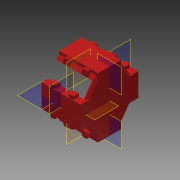
# Autodesk Inventor part: ButtConnector
Saved by Autodesk Inventor 2015 (Build 190159000, 159)
## iProperties
Created: 2015-03-02
Part Number: ButtConnector
Material: Generic
Document SubType Name: Modeling
Designer: Henke
Density: 1 g/cm^3
Appearance: Light Red
Author: Henke
Autodesk Inventor part; units mm, degrees
ref_plane "YZ Plane" through (0, 0, 0) normal (1, 0, 0) x (0, 1, 0)
ref_plane "XZ Plane" through (0, 0, 0) normal (0, 1, 0) x (-1, 0, 0)
ref_plane "XY Plane" through (0, 0, 0) normal (0, 0, 1) x (1, 0, 0)
sketch "Sketch1" plane through (0, 0, 0) normal (0, 0, 1) x (1, 0, 0)
  line L0 (0, 0) -> (35.7, 0)
  line L1 (35.7, 0) -> (35.7, 21.1)
  line L2 (35.7, 21.1) -> (0, 21.1)
  line L3 (0, 21.1) -> (0, 0)
  dimension "d0" = 35.7
  dimension "d1" = 21.1
  constraints: 8 end point, 2 parallel, 1 horizontal, 1 perpendicular
  measures "d0" distance of L1.end L2.end
  measures "d1" distance of L2.end L0.start
extrude "Extrusion1" add sketch "Sketch1" along normal blind 6
sketch "Sketch3" plane through (0, 21.1, 0) normal (0, 1, 0) x (1, 0, 0)
  line L0 (0, 0) -> (35.7, 0) projected
  line L1 (9.35, 0) -> (6.85, -1.05)
  line L2 (6.85, -1.05) -> (6.85, -5.55)
  line L3 (11.85, -5.55) -> (11.85, -1.05)
  line L4 (11.85, -1.05) -> (9.35, 0)
  line L5 (17.85, 0) -> (17.85, -6) construction
  line L6 (6.85, -5.55) -> (11.85, -5.55)
  line L7 (0, -6) -> (35.7, -6) projected
  dimension "d4" = 4.5
  dimension "d5" = 5
  dimension "d6" = 8.5
  dimension "d9" = 5.55
  constraints: 12 end point, 2 equal length, 2 midpoint, 2 vertical, 1 parallel, 1 point on line
  measures "d4" distance of L1.end L2.end
  measures "d5" distance between parallel lines of L3 L2
  measures "d6" distance from line of L5 L1.start
  measures "d9" distance from line of L6 L1.start
extrude "Extrusion2" add sketch "Sketch3" along normal blind 2.75
ref_plane "Work Plane1" through (17.85, 0, 6) normal (1, 0, 0) x (0, 1, 0)
mirror "Mirror1" about plane through (17.85, 0, 6) normal (1, 0, 0) of "Extrusion2"
ref_plane "Work Plane2" through (35.7, 10.55, 6) normal (0, 1, 0) x (-1, 0, 0)
mirror "Mirror2" about plane through (35.7, 10.55, 6) normal (0, 1, 0) of "Extrusion2", "Mirror1"
sketch "Sketch4" plane through (0, 0, 6) normal (0, 0, 1) x (1, 0, 0)
  line L0 (35.7, 21.1) -> (0, 21.1) projected
  line L1 (35.7, 0) -> (32.7, 0)
  line L2 (32.7, 0) -> (32.7, 21.1)
  line L3 (32.7, 21.1) -> (35.7, 21.1)
  line L4 (35.7, 21.1) -> (35.7, 0)
  point P0 (0, 0)
  dimension "d10" = 3
  constraints: 8 end point, 2 parallel, 1 horizontal, 1 perpendicular, 1 point on line
  measures "d10" distance between parallel lines of L4 L2
extrude "Extrusion3" add sketch "Sketch4" along normal blind 21.5
sketch "Sketch6" plane through (0, 0, 6) normal (0, 0, 1) x (1, 0, 0)
  line L0 (32.7, 0) -> (32.7, 21.1) projected
  line L1 (0, 0) -> (32.7, 0)
  line L2 (32.7, 0) -> (32.7, 3)
  line L3 (32.7, 3) -> (0, 3)
  line L4 (0, 3) -> (0, 0)
  line L5 (0, 21.1) -> (32.7, 21.1)
  line L6 (32.7, 21.1) -> (32.7, 18.1)
  line L7 (32.7, 18.1) -> (0, 18.1)
  line L8 (0, 18.1) -> (0, 21.1)
  dimension "d13" = 3
  dimension "d14" = 3
  constraints: 16 end point, 4 parallel, 2 horizontal, 2 perpendicular, 2 point on line
  measures "d13" distance of L7.end L5.start
  measures "d14" distance of L3.end L1.start
mirror "Mirror3" about plane through (34.2, 10.55, 27.5) normal (0, 0, 1) of "Extrusion1", "Extrusion2", "Mirror1", "Mirror2", "Extrusion3"
ref_plane "Work Plane5" through (32.7, 0, 27.5) normal (0, 0, 1) x (1, 0, 0)
sketch "Sketch7" plane through (0, 0, 0) normal (0, -1, 0) x (1, 0, 0)
  line L0 (35.7, 0) -> (35.7, 55) projected
  line L1 (32.7, 6) -> (32.7, 49) projected
  line L2 (35.7, 16.95) -> (32.7, 16.95)
  line L3 (32.7, 16.95) -> (32.7, 38.05)
  line L4 (32.7, 38.05) -> (35.7, 38.05)
  line L5 (35.7, 38.05) -> (35.7, 16.95)
  line L6 (32.7, 6) -> (32.7, 49) projected
  point P0 (0, 0)
  point P1 (32.7, 27.5)
  point P2 (32.7, 27.5)
  dimension "d15" = 21.1
  constraints: 8 end point, 2 midpoint, 2 parallel, 2 point on line, 1 coincident, 1 horizontal, 1 perpendicular
  measures "d15" distance between parallel lines of L4 L2
extrude "Extrusion4" add sketch "Sketch7" along normal blind 10
sketch "Sketch8" plane through (0, -10, 0) normal (0, -1, 0) x (1, 0, 0)
  line L0 (32.7, 38.05) -> (35.7, 38.05) projected
  line L1 (35.7, 38.05) -> (35.7, 16.95) projected
  line L2 (35.7, 16.95) -> (32.7, 16.95) projected
  line L3 (32.7, 16.95) -> (32.7, 38.05) projected
  line L4 (35.7, 16.95) -> (0, 16.95)
  line L5 (0, 16.95) -> (0, 38.05)
  line L6 (0, 38.05) -> (35.7, 38.05)
  line L7 (35.7, 38.05) -> (35.7, 16.95)
  point P0 (0, 0)
  dimension "d18" = 35.7
  constraints: 8 end point, 2 parallel, 1 horizontal, 1 perpendicular
  measures "d18" distance of L5.end L0.end
extrude "Extrusion5" add sketch "Sketch8" along normal blind 6
sketch "Sketch9" plane through (35.7, 0, 16.95) normal (0, 0, -1) x (-1, 0, 0)
  line L0 (35.7, -16) -> (0, -16) projected
  line L1 (26.35, -16) -> (28.85, -14.95)
  line L2 (28.85, -14.95) -> (28.85, -10.45)
  line L3 (28.85, -10.45) -> (23.85, -10.45)
  line L4 (23.85, -10.45) -> (23.85, -14.95)
  line L5 (23.85, -14.95) -> (26.35, -16)
  line L6 (17.85, -16) -> (17.85, -10) construction
  line L7 (35.7, -10) -> (3, -10) construction
  point P0 (35.7, 0)
  dimension "d21" = 4.5
  dimension "d22" = 5.55
  dimension "d23" = 8.5
  dimension "d24" = 5
  constraints: 12 end point, 3 perpendicular, 2 equal length, 2 point on line, 1 midpoint, 1 vertical
  measures "d21" distance of L1.end L2.end
  measures "d22" distance from line of L3 L1.start
  measures "d23" distance from line of L6 L1.start
  measures "d24" distance between parallel lines of L4 L2
extrude "Extrusion6" add sketch "Sketch9" along normal blind 2.75
ref_plane "Work Plane6" through (0, -16, 27.5) normal (0, 0, -1) x (-1, 0, 0)
ref_plane "Work Plane7" through (17.85, -16, 38.05) normal (-1, 0, 0) x (0, -1, 0)
mirror "Mirror4" about plane through (17.85, -16, 38.05) normal (-1, 0, 0) of "Extrusion6"
mirror "Mirror5" about plane through (0, -16, 27.5) normal (0, 0, -1) of "Extrusion6", "Mirror4"
sketch "Sketch10" plane through (0, -10, 0) normal (0, 1, 0) x (1, 0, 0)
  line L0 (32.7, -6) -> (32.7, -49) projected
  line L1 (0, -16.95) -> (32.7, -16.95)
  line L2 (32.7, -16.95) -> (32.7, -20.95)
  line L3 (32.7, -20.95) -> (0, -20.95)
  line L4 (0, -20.95) -> (0, -16.95)
  point P0 (0, 0)
  dimension "d27" = 4
  constraints: 8 end point, 2 parallel, 1 horizontal, 1 perpendicular, 1 point on line
  measures "d27" distance of L3.end L1.start
chamfer "Chamfer2" distance 14.45 distance2 10 1 edges at (34.2, 0, 16.95) measured on face at (34.2, 0, 16.45)
loft "Loft1" [suppressed]
chamfer "Chamfer4" distance 14.45 distance2 10 1 edges at (34.2, 0, 38.05) measured on face at (34.2, 0, 38.55)
mirror "Mirror6" [suppressed]
chamfer "Chamfer3" distance 2 angle 45 2 edges at (35.7, -5, 9.725) (35.7, -5, 45.275)
mirror "Mirror7" about plane through (35.7, 10.55, 6) normal (0, 1, 0) of "Extrusion4", "Extrusion5", "Extrusion6", "Mirror4", "Mirror5"
chamfer "Chamfer5" distance 14.45 distance2 10 1 edges at (34.2, 21.1, 16.95) measured on face at (34.2, 21.1, 16.45)
chamfer "Chamfer6" distance 14.45 distance2 10 1 edges at (34.2, 21.1, 38.05) measured on face at (34.2, 21.1, 38.55)
mirror "Mirror8" [suppressed]
chamfer "Chamfer7" distance 2 angle 45 2 edges at (35.7, 26.1, 45.275) (35.7, 26.1, 9.725)
ref_plane "Work Plane3" through (17.85, 0, 49) normal (-1, 0, 0) x (0, 1, 0)
ref_plane "Work Plane4" through (35.7, 10.55, 49) normal (0, -1, 0) x (-1, 0, 0)
ref_plane "Work Plane8" through (17.85, 37.1, 38.05) normal (1, 0, 0) x (0, 1, 0)
ref_plane "Work Plane9" through (0, 37.1, 27.5) normal (0, 0, 1) x (-1, 0, 0)
body "Solid1"
